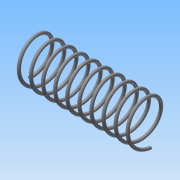
# Autodesk Inventor part: пружинка  концевика
Saved by Autodesk Inventor 2017 (Build 210142000, 142)
## iProperties
Part Number: пружинка  концевика
Material: Типовые
Document SubType Name: Modeling
Designer: Max
Mass: 0.0500596 g
Surface Area: 4.05918 cm^2
Volume: 0.0500596 cm^3
Density: 1 g/cm^3
Appearance: Сталь - гальванизированная
Author: Max
Autodesk Inventor part; units mm, degrees
ref_plane "YZ Plane" through (0, 0, 0) normal (1, 0, 0) x (0, 1, 0)
ref_plane "XZ Plane" through (0, 0, 0) normal (0, 1, 0) x (-1, 0, 0)
ref_plane "XY Plane" through (0, 0, 0) normal (0, 0, 1) x (1, 0, 0)
sketch "Эскиз1" plane through (0, 0, 0) normal (0, 1, 0) x (-1, 0, 0)
  line L0 (0, 0) -> (36.6922, 0)
  circle A0 centre (0, -3.25) radius 0.25
  dimension "d0" = 0.5
  dimension "d1" = 3
  constraints: 2 end point, 1 centre point, 1 horizontal
  measures "d0" diameter of A0
  measures "d1" distance edge to line of A0 L0
coil "Пружина1" sketch "Эскиз1" operation add axis through (0, 0, 0) along (-1, 0, 0) pitch 2 turns 20 hand right
sketch "Эскиз2" plane through (0, 0, 0) normal (0, 0, 1) x (1, 0, 0)
  line L0 (-3.8534, 9.9624) -> (6.485, 9.9624)
  line L1 (6.485, 9.9624) -> (6.485, -5.9211)
  line L2 (6.485, -5.9211) -> (-3.8534, -5.9211)
  line L3 (-3.8534, -5.9211) -> (-3.8534, 9.9624)
  line L4 (-42.3872, 15.5075) -> (-28.8534, 15.5075)
  line L5 (-28.8534, 15.5075) -> (-28.8534, -7.6128)
  line L6 (-28.8534, -7.6128) -> (-42.3872, -7.6128)
  line L7 (-42.3872, -7.6128) -> (-42.3872, 15.5075)
  point P0 (0, 0)
  dimension "d10" = 25
  constraints: 16 end point, 4 parallel, 2 horizontal, 2 perpendicular
  measures "d10" distance between parallel lines of L3 L5
extrude "Выдавливание1" cut sketch "Эскиз2" along normal mid plane 20
